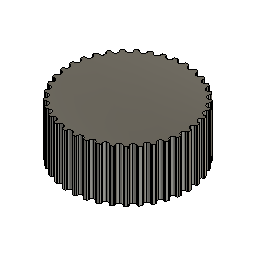
gear_37z (Autodesk Fusion 360 design; units mm, degrees)
Autodesk Fusion 360 part; units mm, degrees
sketch "Sketch1" plane through (0, 0, 0) normal (0, 0, 1) x (1, 0, 0) in component "gt2 pulley"
  circle A0 centre (0, 0) radius 11.7775 construction
  circle A1 centre (0, 0) radius 10.7735 construction
  line L0 (0, 0) -> (0, 11.7775) construction
  line L1 (0, 0) -> (0.9988, 11.735) construction
  line L2 (0, 0) -> (1.409, 11.6929) construction
  circle A2 centre (0, 0) radius 11.5235 construction
  arc A3 (0.3804, 11.3802) -> (0.4396, 11.0968) centre (1.3786, 11.4407) ccw
  circle A4 centre (0, 0) radius 11.3735 construction
  arc A5 (0.2337, 11.5211) -> (0, 11.5235) centre (0, 0) ccw
  arc A6 (0.3804, 11.3802) -> (0.2337, 11.5211) centre (0.2307, 11.3711) ccw
  arc A7 (0.4396, 11.0968) -> (0.9137, 10.7347) centre (0.9607, 11.2877) ccw
  arc A8 (0, 11.5235) -> (-0.2337, 11.5211) centre (0, 0) ccw
  arc A9 (-0.2337, 11.5211) -> (-0.3804, 11.3802) centre (-0.2307, 11.3711) ccw
  arc A10 (-0.4396, 11.0968) -> (-0.3804, 11.3802) centre (-1.3786, 11.4407) ccw
  arc A11 (-0.9137, 10.7347) -> (-0.4396, 11.0968) centre (-0.9607, 11.2877) ccw
  arc A12 (0.9137, 10.7347) -> (-0.9137, 10.7347) centre (0, 0) ccw
  point P0 (1.3786, 11.4407)
  point P1 (0, 11.5235)
  dimension "d18" = 23.5549
  dimension "d19" = 4.865
  dimension "d22" = 1.004
  dimension "d24" = 0.75
  dimension "d26" = 1
  dimension "d27" = 0.15
  dimension "d28" = 0.15
  dimension "d47" = 0.555
  dimension "d52" = 3.812
  constraint coincident A0.centre A1.centre
  constraint coincident A0 L0.end
  constraint vertical L0
  constraint coincident A0 L1.end
  constraint coincident A0 L2.end
  constraint concentric A1 A2
  constraint coincident A1 A7.end
  constraint coincident L1 A7.end
  constraint coincident A2 P0
  constraint coincident L2 P0
  constraint coincident P0 A3.centre
  constraint coincident A2 P1
  constraint coincident L0 P1
  constraint concentric A2 A4
  constraint coincident P1 A5.end
  constraint coincident A4 A6.centre
  constraint coincident A3.start A6.start
  constraint tangent A3 A6
  constraint tangent A3 A7
  constraint symmetric L0 A7.end A11.start
  constraint symmetric L0 A3.start A9.end
  constraint symmetric L0 A3.end A10.start
  constraint symmetric L0 A3 A10
  constraint symmetric L0 A5.start A8.end
  constraint symmetric L0 P1 A5.end
  constraint symmetric L0 A5 A8
  constraint symmetric L0 A6 A9
  constraint symmetric L0 A7 A11
  constraint coincident A1 A11.start
  constraint tangent A1 A7
  constraint coincident L1 A7.centre
  measures "d18" diameter of A0
  measures "d19" angle of L0 L1
  measures "d22" distance of A0 A1
  measures "d24" distance of A1 A2
  measures "d26" radius of A3
  measures "d27" distance of A2 A4
  measures "d28" radius of A6
  measures "d47" radius of A7
extrude "Extrude1" add sketch "Sketch1" along normal blind 10 makes body 1
pattern_circular "C-Pattern1" count 37 over 360 about axis through (0, 0, 1.75) along (0, 0, 1) of bodies 1 makes body 2 at (-1.9208, 10.6008, 6.6667) makes body 3 at (-4.2516, 9.8991, 6.6667) makes body 4 at (-4.622, 9.7316, 3.3333) makes body 5 at (-6.8469, 8.3179, 6.6667) makes body 6 at (-7.6, 7.6359, 3.3333) makes body 7 at (-9.5267, 5.0309, 6.6667) makes body 8 at (-9.7097, 4.6679, 3.3333) makes body 9 at (-10.6585, 1.5698, 6.6667) makes body 10 at (-10.7705, -0.2541, 6.6667) makes body 11 at (-10.5726, -2.0706, 6.6667) makes body 12 at (-10.487, -2.468, 3.3333) makes body 13 at (-9.2789, -5.4745, 6.6667) makes body 14 at (-8.2202, -6.9639, 6.6667) makes body 15 at (-7.3809, -7.848, 6.6667) makes body 16 at (-6.6088, -8.5083, 3.3333) makes body 17 at (-5.0758, -9.5028, 3.3333) makes body 18 at (-3.3968, -10.224, 3.3333) makes body 19 at (-0.2033, -10.7715, 6.6667) makes body 20 at (1.6201, -10.651, 6.6667) makes body 21 at (2.8129, -10.3998, 6.6667) makes body 22 at (5.0758, -9.5028, 6.6667) makes body 23 at (6.1168, -8.8686, 6.6667) makes body 24 at (6.9251, -8.253, 3.3333) makes body 25 at (8.2202, -6.9639, 3.3333) makes body 26 at (9.2789, -5.4745, 3.3333) makes body 27 at (10.3305, -3.0574, 6.6667) makes body 28 at (10.5726, -2.0706, 3.3333) makes body 29 at (10.7101, 1.1666, 6.6667) makes body 30 at (10.3589, 2.9598, 6.6667) makes body 31 at (10.2399, 3.3485, 3.3333) makes body 32 at (9.5267, 5.0309, 3.3333) makes body 33 at (7.6, 7.6359, 6.6667) makes body 34 at (7.3065, 7.9172, 3.3333) makes body 35 at (5.1652, 9.4545, 6.6667) makes body 36 at (4.2516, 9.8991, 3.3333) makes body 37 at (2.5175, 10.4752, 3.3333)
sketch "Sketch2" plane through (0, 0, 10) normal (0, 0, 1) x (-1, 0, 0)
  arc A0 (-11.3861, -0.1029) -> (-11.5206, -0.2555) centre (-11.3707, -0.2521) ccw
  arc A1 (-11.5206, -0.2555) -> (-11.5008, -0.7224) centre (0, 0) ccw
  arc A2 (-11.5008, -0.7224) -> (-11.3538, -0.8631) centre (-11.3511, -0.7131) ccw
  arc A3 (-11.0681, -0.9101) -> (-11.3538, -0.8631) centre (-11.3719, -1.8629) ccw
  arc A4 (-10.6862, -1.3684) -> (-11.0681, -0.9101) centre (-11.2367, -1.4389) ccw
  arc A5 (-10.7638, 0.4572) -> (-10.6862, -1.3684) centre (0, 0) ccw
  arc A6 (-11.1054, -0.0318) -> (-10.7638, 0.4572) centre (-11.3183, 0.4808) ccw
  arc A7 (-11.3861, -0.1029) -> (-11.1054, -0.0318) centre (-11.4889, 0.8918) ccw
  circle A8 centre (0, 0) radius 10.7735
  constraint coincident A1.centre A5.centre
extrude "Extrude2" add sketch "Sketch2" against normal blind 10 contours A5 A8 bodies 1 2 3 4 5 6 7 8 9 10 11 12 13 14 15 16 17 18 19 20 21 22 23 24 25 26 27 28 29 30 31 32 33 34 35 36 37
extrude "Extrude4" [suppressed] in component "gt2 pulley"
pattern_circular "C-Pattern7" [suppressed] in component "gt2 pulley"
extrude "Extrude3" [suppressed] in component "gt2 pulley"
pattern_circular "C-Pattern6" [suppressed] in component "gt2 pulley"
extrude "Extrude2'" [suppressed] in component "gt2 pulley"
pattern_circular "C-Pattern5" [suppressed] in component "gt2 pulley"
extrude "Extrude1'" [suppressed] in component "gt2 pulley"
pattern_circular "C-Pattern4" [suppressed] in component "gt2 pulley"
pattern_circular "C-Pattern3" [suppressed] in component "gt2 pulley"
pattern_circular "C-Pattern2" [suppressed] in component "gt2 pulley"
pattern_circular "C-Pattern1'" [suppressed] in component "gt2 pulley"
copy_body "Body->Comp1" [suppressed] in component "Component"
copy_body "Body->Comp2" [suppressed] in component "Component'"
copy_body "Body->Comp3" [suppressed] in component "Component''"
copy_body "Body->Comp4" [suppressed] in component "Component'''"
copy_body "Body->Comp5" [suppressed] in component "Component''''"
copy_body "Body->Comp6" [suppressed] in component "Component'''''"
copy_body "Body->Comp7" [suppressed] in component "Component''''''"
copy_body "Body->Comp8" [suppressed] in component "Component'''''''"
copy_body "Body->Comp9" [suppressed] in component "Component''''''''"
copy_body "Body->Comp10" [suppressed] in component "Component'''''''''"
copy_body "Body->Comp11" [suppressed] in component "Component''''''''''"
copy_body "Body->Comp12" [suppressed] in component "Component'''''''''''"
copy_body "Body->Comp13" [suppressed] in component "Component''''''''''''"
copy_body "Body->Comp14" [suppressed] in component "Component'''''''''''''"
copy_body "Body->Comp15" [suppressed] in component "Component''''''''''''''"
copy_body "Body->Comp16" [suppressed] in component "Component'''''''''''''''"
copy_body "Body->Comp17" [suppressed] in component "Component''''''''''''''''"
copy_body "Body->Comp18" [suppressed] in component "Component'''''''''''''''''"
copy_body "Body->Comp19" [suppressed] in component "Component''''''''''''''''''"
copy_body "Body->Comp20" [suppressed] in component "Component'''''''''''''''''''"
component "gt2 pulley" placed x (1, 0, 0) y (0, 1, 0) z (0, 0, 1) at (0, 0, 0)
equation "NumTeeth = 37" comment "min 20"
equation "ToothPitch = 2 mm"
equation "PullyDia = NumTeeth * ToothPitch / PI"
equation "ToothAng = ( ( 360 / NumTeeth ) * 1 deg )"
equation "TransOffsetAngle = ToothAng * 0.2"
equation "Sholulder_Radius = 0.15 mm"
equation "Root_Radius = 0.555 mm"
equation "TransRadius = 1 mm"
equation "ToolHeight = 0.75 mm"
equation "PLD = 0.254 mm"
equation "d18 = PullyDia"
equation "d19 = ToothAng / 2"
equation "d22 = PLD + ToolHeight"
equation "d24 = ToolHeight"
equation "d26 = TransRadius"
equation "d27 = Sholulder_Radius"
equation "d31 = NumTeeth"
equation "d33 = NumTeeth"
equation "d35 = NumTeeth"
equation "d37 = NumTeeth"
equation "d41 = NumTeeth"
equation "d45 = NumTeeth"
equation "d47 = Root_Radius"
equation "d50 = NumTeeth"
